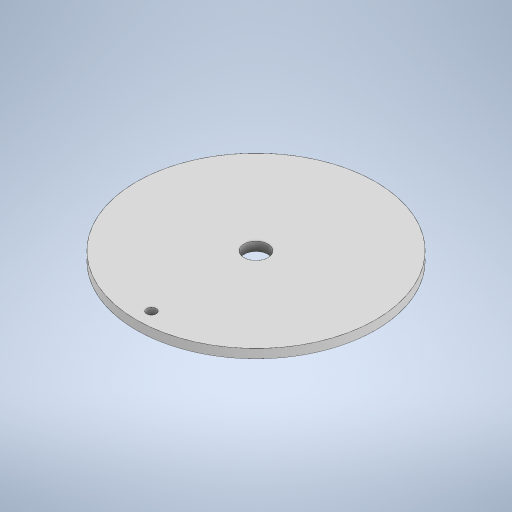
# Autodesk Inventor part: NHK_t0_2
Saved by Autodesk Inventor 2023 (Build 270158000, 158)
## iProperties
Created: 2022-04-18
Part Number: NHK_t0_2
Material: 一般
Document SubType Name: Modeling
Designer: yuta
Density: 1 g/cm^3
Appearance: 既定
Author: yuta
Autodesk Inventor part; units mm, degrees
ref_plane "YZ Plane" through (0, 0, 0) normal (1, 0, 0) x (0, 1, 0)
ref_plane "XZ Plane" through (0, 0, 0) normal (0, 1, 0) x (-1, 0, 0)
ref_plane "XY Plane" through (0, 0, 0) normal (0, 0, 1) x (1, 0, 0)
sketch "スケッチ1" plane through (0, 0, 0) normal (0, 1, 0) x (-1, 0, 0)
  circle A0 centre (0, 0) radius 40
  dimension "d0" = 80
  constraints: 1 centre point, 1 coincident
  measures "d0" diameter of A0
extrude "押し出し1" add sketch "スケッチ1" along normal blind 3
sketch "スケッチ2" plane through (0, 3, 0) normal (0, 1, 0) x (1, 0, 0)
  circle A0 centre (0, 0) radius 4
  dimension "d3" = 8
  constraints: 1 centre point, 1 coincident
  measures "d3" diameter of A0
extrude "押し出し2" cut sketch "スケッチ2" against normal blind 3
sketch "スケッチ3" plane through (0, 3, 0) normal (0, 1, 0) x (1, 0, 0)
  circle A0 centre (0, -35) radius 1.6
  circle A1 centre (0, 0) radius 40 projected
  dimension "d6" = 3.2
  dimension "d7" = 35
  constraints: 1 centre point
  measures "d6" diameter of A0
  measures "d7" distance of A1.centre A0.centre
hole "穴1" at (0, 3, 35) direction (0, -1, 0) diameter 3.2 end through all
